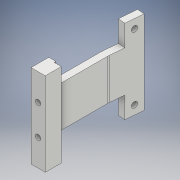
# Autodesk Inventor part: 대각선PSD받침대
Saved by Autodesk Inventor 2017 (Build 210142000, 142)
## iProperties
Part Number: 대각선PSD받침대
Material: ABS 플라스틱
Document SubType Name: Modeling
Designer: minom
Density: 1.06 g/cm^3
Appearance: 매끄러움 - 흰색
Mass: 8.45301 g
Surface Area: 50.9434 cm^2
Volume: 7.97454 cm^3
Author: minom
Autodesk Inventor part; units mm, degrees
ref_plane "YZ Plane" through (0, 0, 0) normal (1, 0, 0) x (0, 1, 0)
ref_plane "XZ Plane" through (0, 0, 0) normal (0, 1, 0) x (-1, 0, 0)
ref_plane "XY Plane" through (0, 0, 0) normal (0, 0, 1) x (1, 0, 0)
sketch "스케치1" plane through (0, 0, 0) normal (1, 0, 0) x (0, 1, 0)
  line L0 (0, 0) -> (55, 0)
  line L1 (55, 0) -> (55, -47)
  line L2 (55, -47) -> (0, -47)
  line L3 (0, -47) -> (0, 0)
  circle A0 centre (50, -5) radius 1.6
  circle A1 centre (50, -42) radius 1.6
  dimension "d0" = 55
  dimension "d1" = 47
  dimension "d2" = 3.2
  dimension "d3" = 3.2
  dimension "d4" = 50
  dimension "d5" = 50
  dimension "d6" = 5
  dimension "d7" = 5
  constraints: 8 end point, 2 centre point, 2 parallel, 1 horizontal, 1 perpendicular
  measures "d0" distance of L1.end L2.end
  measures "d1" distance of L0.end L1.end
  measures "d2" diameter of A0
  measures "d3" diameter of A1
  measures "d4" distance from line of A0.centre L3
  measures "d5" distance from line of L3 A1.centre
  measures "d6" distance from line of L0 A0.centre
  measures "d7" distance from line of L2 A1.centre
extrude "돌출1" add sketch "스케치1" along normal blind 8
sketch "스케치2" plane through (8, 0, 0) normal (1, 0, 0) x (0, 0, -1)
  circle A0 centre (42, 50) radius 1.6 projected
  circle A1 centre (5, 50) radius 1.6 projected
  line L0 (0, 55) -> (0, 0) projected
  line L1 (0, 0) -> (47, 0) projected
  line L2 (47, 0) -> (47, 55) projected
  line L3 (47, 55) -> (0, 55) projected
  line L4 (47, 0) -> (47, 55) projected
  line L5 (0, 0) -> (47, 0)
  line L6 (47, 0) -> (47, 6)
  line L7 (47, 6) -> (0, 6)
  line L8 (0, 6) -> (0, 0)
  dimension "d10" = 6
  constraints: 8 end point, 2 parallel, 1 horizontal, 1 perpendicular, 1 point on line
  measures "d10" distance between parallel lines of L7 L1
extrude "돌출2" cut sketch "스케치2" against normal blind 4 contours L3 L2 L7 L0
sketch "스케치3" plane through (4, 0, 0) normal (1, 0, 0) x (0, 0, -1)
  line L0 (47, 6) -> (0, 6) projected
  line L1 (47, 55) -> (47, 6) projected
  line L2 (0, 55) -> (47, 55) projected
  line L3 (0, 6) -> (0, 55) projected
  circle A0 centre (42, 50) radius 1.6 projected
  circle A1 centre (5, 50) radius 1.6 projected
  line L4 (0, 0) -> (0, 55) projected
  line L5 (47, 6) -> (0, 6) projected
  line L6 (47, 55) -> (47, 0) projected
  line L7 (12, 45) -> (12, 7)
  line L8 (35, 45) -> (35, 7)
  line L9 (0, 7) -> (12, 7)
  line L10 (35, 7) -> (47, 7)
  line L11 (0, 45) -> (12, 45)
  line L12 (35, 45) -> (47, 45)
  dimension "d17" = 12
  dimension "d18" = 12
  dimension "d19" = 38
  dimension "d20" = 38
  dimension "d21" = 1
  dimension "d22" = 1
  constraints: 12 end point, 8 perpendicular, 4 point on line
  measures "d17" distance between parallel lines of L7 L3
  measures "d18" distance between parallel lines of L1 L8
  measures "d19" distance between parallel lines of L9 L11
  measures "d20" distance between parallel lines of L12 L10
  measures "d21" distance between parallel lines of L0 L9
  measures "d22" distance between parallel lines of L0 L10
extrude "돌출3" cut sketch "스케치3" against normal blind 4 contours L10 L8 L12 L1 | L3 L11 L7 L9
sketch "스케치4" plane through (0, 0, -47) normal (0, -1, 0) x (1, 0, 0)
  line L0 (0, 0) -> (0, 47) projected
  line L1 (0, 0) -> (8, 0) projected
  line L2 (8, 47) -> (8, 0) projected
  line L3 (0, 47) -> (8, 47) projected
  circle A0 centre (4, 32) radius 1.5
  circle A1 centre (4, 15) radius 1.5
  dimension "d25" = 3
  dimension "d26" = 3
  dimension "d27" = 4
  dimension "d28" = 4
  dimension "d29" = 15
  dimension "d30" = 15
  constraints: 2 centre point
  measures "d25" diameter of A0
  measures "d26" diameter of A1
  measures "d27" distance from line of L0 A0.centre
  measures "d28" distance from line of L0 A1.centre
  measures "d29" distance from line of L3 A0.centre
  measures "d30" distance from line of L1 A1.centre
extrude "돌출4" cut sketch "스케치4" against normal blind 3 contours A0 | A1
sketch "스케치6" plane through (4, 0, 0) normal (1, 0, 0) x (0, 0, -1)
  circle A0 centre (5, 50) radius 1.6 projected
  circle A1 centre (42, 50) radius 1.6 projected
  line L0 (47, 6) -> (0, 6) projected
  line L1 (47, 7) -> (47, 6) projected
  line L2 (47, 7) -> (35, 7) projected
  line L3 (35, 7) -> (35, 45) projected
  line L4 (35, 45) -> (47, 45) projected
  line L5 (47, 55) -> (47, 45) projected
  line L6 (0, 55) -> (47, 55) projected
  line L7 (0, 45) -> (0, 55) projected
  line L8 (0, 45) -> (12, 45) projected
  line L9 (12, 45) -> (12, 7) projected
  line L10 (12, 7) -> (0, 7) projected
  line L11 (0, 6) -> (0, 7) projected
  line L12 (12, 45) -> (12, 7) projected
  line L13 (12, 36) -> (35, 36)
  point P0 (0, 0)
  dimension "d39" = 30
  constraints: 2 end point, 2 point on line, 1 perpendicular
  measures "d39" distance between parallel lines of L13 L0
bend part "굽힘1" radius 10 angle 5 line through (4, 36, -12) along (0, 0, -1) centre toward (1, 0, 0) moving side (0, 1, 0) both sides no
sketch "스케치8" plane through (0, 0, -47) normal (0, -1, 0) x (1, 0, 0)
  circle A0 centre (4, 32) radius 1.5 projected
  circle A1 centre (4, 15) radius 1.5 projected
  line L0 (0, 0) -> (0, 47) projected
  line L1 (0, 0) -> (8, 0) projected
  line L2 (8, 47) -> (8, 0) projected
  line L3 (0, 47) -> (8, 47) projected
extrude "돌출7" add sketch "스케치8" along normal blind 3
